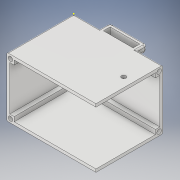
# Autodesk Inventor part: Part3
Saved by Autodesk Inventor 2019 (Build 230136000, 136)
## iProperties
Created: 2019-02-07
Part Number: Part3
Material: ABS Plastic
Document SubType Name: Modeling
Designer: darky
Density: 1.06 g/cm^3
Appearance: Smooth - White
Author: darky
Autodesk Inventor part; units mm, degrees
ref_plane "YZ Plane" through (0, 0, 0) normal (1, 0, 0) x (0, 1, 0)
ref_plane "XZ Plane" through (0, 0, 0) normal (0, 1, 0) x (-1, 0, 0)
ref_plane "XY Plane" through (0, 0, 0) normal (0, 0, 1) x (1, 0, 0)
sketch "Sketch2" plane through (0, 0, 0) normal (0, 0, 1) x (1, 0, 0)
  line L0 (0, 0) -> (60, 0)
  line L1 (60, 0) -> (60, 40)
  line L2 (60, 40) -> (0, 40)
  line L3 (0, 40) -> (0, 0)
  dimension "d11" = 60
  dimension "d12" = 40
  constraints: 8 end point, 2 parallel, 1 horizontal, 1 perpendicular
  measures "d11" distance of L2.end L1.end
  measures "d12" distance of L1.end L0.end
extrude "Extrusion1" add sketch "Sketch2" along normal blind 45
shell "Shell1" thickness 5 removed faces 2 at (20, 26.6667, 45) at (60, 13.3333, 30)
sketch "Sketch4" plane through (0, 0, 45) normal (0, 0, 1) x (1, 0, 0)
  line L0 (5, 35) -> (5, 5) projected
  circle A0 centre (2.4749, 37.4236) radius 2
  circle A1 centre (2.4749, 2.5764) radius 2
  point P0 (0, 0)
  dimension "d20" = 4
  dimension "d21" = 4
  constraints: 2 centre point
  measures "d20" diameter of A0
  measures "d21" diameter of A1
hole "Hole2" at (2.4749, 37.4236, 45) direction (0, 0, -1) diameter 3 depth 9 tip angle 118
sketch "Sketch6" plane through (0, 0, 45) normal (0, 0, 1) x (1, 0, 0)
  line L0 (5, 35) -> (5, 5) projected
  circle A0 centre (2.5251, 2.5251) radius 2
  point P0 (0, 0)
  dimension "d37" = 4
  constraints: 1 centre point
  measures "d37" diameter of A0
hole "Hole3" at (2.5251, 2.5251, 45) direction (0, 0, -1) diameter 3 depth 9 tip angle 118
sketch "Sketch7" plane through (60, 0, 0) normal (1, 0, 0) x (0, 0, -1)
  line L0 (-5, 35) -> (-45, 35) projected
  circle A0 centre (-2.5251, 37.4749) radius 2
  point P0 (0, 0)
  dimension "d46" = 4
  constraints: 1 centre point
  measures "d46" diameter of A0
hole "Hole4" at (60, 37.4749, 2.5251) direction (-1, 0, 0) diameter 3 depth 9 tip angle 118
sketch "Sketch8" plane through (60, 0, 0) normal (1, 0, 0) x (0, 0, -1)
  line L0 (-5, 35) -> (-5, 5) projected
  circle A0 centre (-2.5251, 2.5251) radius 2
  point P0 (0, 0)
  dimension "d55" = 4
  constraints: 1 centre point
  measures "d55" diameter of A0
hole "Hole5" at (60, 2.5251, 2.5251) direction (-1, 0, 0) diameter 3 depth 9 tip angle 118
sketch "Sketch11" plane through (0, 0, 45) normal (0, 0, 1) x (1, 0, 0)
  line L0 (60, 35) -> (5, 35) projected
  line L1 (60, 38.9749) -> (60, 35.9749) projected
  line L2 (5, 35) -> (60, 35)
  line L3 (60, 35) -> (60, 38)
  line L4 (60, 38) -> (5, 38)
  line L5 (5, 38) -> (5, 35)
  point P0 (0, 0)
  dimension "d76" = 3
  constraints: 8 end point, 2 parallel, 1 horizontal, 1 perpendicular, 1 point on line
  measures "d76" distance of L3.end L2.end
extrude "Extrusion4" cut sketch "Sketch11" against normal blind 40
sketch "Sketch12" plane through (0, 0, 45) normal (0, 0, 1) x (1, 0, 0)
  line L0 (5, 38) -> (5, 5) projected
  line L1 (60, 4.0251) -> (60, 1.0251) projected
  line L2 (5, 5) -> (60, 5)
  line L3 (60, 5) -> (60, 2)
  line L4 (60, 2) -> (5, 2)
  line L5 (5, 2) -> (5, 5)
  point P0 (0, 0)
  dimension "d79" = 3
  constraints: 8 end point, 2 parallel, 1 horizontal, 1 perpendicular, 1 point on line
  measures "d79" distance of L2.end L3.end
extrude "Extrusion5" cut sketch "Sketch12" against normal blind 40
sketch "Sketch13" plane through (0, 0, 45) normal (0, 0, 1) x (1, 0, 0)
  line L0 (5, 38) -> (60, 38) projected
  line L1 (5, 38) -> (5, 35)
  line L2 (5, 2) -> (5, 38) projected
  line L3 (5, 35) -> (2, 35)
  line L4 (2, 35) -> (2, 5)
  line L5 (2, 5) -> (5, 5)
  line L6 (5, 5) -> (5, 35)
  point P0 (0, 0)
  dimension "d82" = 3
  dimension "d83" = 3
  dimension "d84" = 30
  constraints: 10 end point, 2 parallel, 1 horizontal, 1 perpendicular, 1 point on line
  measures "d82" distance of L0.start L1.end
  measures "d83" distance of L5.end L4.end
  measures "d84" distance of L4.end L3.end
extrude "Extrusion6" cut sketch "Sketch13" against normal blind 40
sketch "Sketch14" plane through (60, 0, 0) normal (1, 0, 0) x (0, 0, -1)
  line L0 (-5, 38) -> (-5, 2) projected
  line L1 (-5, 38) -> (-5, 35)
  line L2 (-5, 35) -> (-2, 35)
  line L3 (-2, 35) -> (-2, 5)
  line L4 (-2, 5) -> (-5, 5)
  line L5 (-5, 5) -> (-5, 35)
  point P0 (0, 0)
  dimension "d87" = 3
  dimension "d88" = 3
  dimension "d89" = 30
  constraints: 10 end point, 2 parallel, 1 horizontal, 1 perpendicular, 1 point on line
  measures "d87" distance of L0.start L1.end
  measures "d88" distance of L3.end L4.end
  measures "d89" distance of L2.end L3.end
extrude "Extrusion7" cut sketch "Sketch14" against normal blind 58
sketch "Sketch18" plane through (5, 38, 45) normal (0, -1, 0) x (1, 0, 0)
  line L0 (0, -40) -> (55, -40) projected
  line L1 (55, -40) -> (55, -25)
  line L2 (55, 0) -> (55, -40) projected
  line L3 (55, -25) -> (49, -25)
  circle A0 centre (48.7205, -25) radius 1.5
  point P0 (-5, -45)
  dimension "d108" = 15
  dimension "d109" = 6
  dimension "d110" = 3
  constraints: 4 end point, 1 centre point, 1 perpendicular, 1 point on line
  measures "d108" distance of L0.end L1.end
  measures "d109" distance of L1.end L3.end
  measures "d110" diameter of A0
extrude "Extrusion10" cut sketch "Sketch18" against normal blind 2
sketch "Sketch19" plane through (0, 0, 0) normal (0, 0, -1) x (-1, 0, 0)
  line L0 (0, 0) -> (0, 40)
  line L1 (0, 40) -> (-30, 40)
  line L2 (-2, 40) -> (-60, 40) projected
  line L3 (-30, 40) -> (-17.5, 40)
  line L4 (-17.5, 40) -> (-42.5, 40)
  line L5 (-42.5, 40) -> (-42.5, 35)
  line L6 (-42.5, 35) -> (-17.5, 35)
  line L7 (-17.5, 35) -> (-17.5, 40)
  dimension "d113" = 40
  dimension "d114" = 30
  dimension "d115" = 12.5
  dimension "d116" = 25
  dimension "d117" = 5
  constraints: 14 end point, 2 parallel, 2 point on line, 1 horizontal, 1 perpendicular, 1 vertical
  measures "d113" distance of L0.start L0.end
  measures "d114" distance of L0.end L1.end
  measures "d115" distance of L1.end L3.end
  measures "d116" distance of L6.end L5.end
  measures "d117" distance of L5.end L4.end
extrude "Extrusion11" add sketch "Sketch19" along normal blind 7
sketch "Sketch20" plane through (0, 40, 45) normal (0, 1, 0) x (1, 0, 0)
  line L0 (42.5, 45) -> (40, 45)
  line L1 (17.5, 45) -> (42.5, 45) projected
  line L2 (40, 45) -> (20, 45)
  line L3 (20, 45) -> (20, 49.5)
  line L4 (20, 49.5) -> (40, 49.5)
  line L5 (40, 49.5) -> (40, 45)
  point P0 (0, 45)
  dimension "d120" = 2.5
  dimension "d121" = 20
  dimension "d122" = 4.5
  constraints: 10 end point, 2 parallel, 1 horizontal, 1 perpendicular, 1 point on line
  measures "d120" distance of L0.start L0.end
  measures "d121" distance of L3.end L4.end
  measures "d122" distance of L2.end L3.end
extrude "Extrusion12" cut sketch "Sketch20" against normal blind 5
fillet "Fillet3" radius 1 9 edges at (51.25, 40, 0) (42.5, 40, -3.5) (30, 40, -7) (17.5, 40, -3.5) (8.75, 40, 0) (0, 40, 22.5) (0, 20, 0) (30, 0, 0) (0, 0, 22.5)
fillet "Fillet4" radius 2 7 edges at (42.2071, 39.7071, -6.7071) (42.5, 37, -7) (30, 35, -7) (17.5, 37, -7) (17.7929, 39.7071, -6.7071) (42.5, 35, -3.5) (17.5, 35, -3.5)
sketch "Sketch21" plane through (1, 40, 45) normal (0, 1, 0) x (1, 0, 0)
  point P0 (-1, 45)
body "Solid1"
